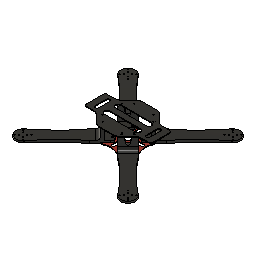
drone-model (Autodesk Fusion 360 design; units mm, degrees)
part number: 2026-04-12-16-53-26-750
Autodesk Fusion 360 part; units mm, degrees
sketch "Sketch1" plane through (0, 0, 0) normal (0, 0, 1) x (1, 0, 0)
  line L0 (-24, 54) -> (24, 54)
  line L1 (54, 24) -> (54, -24)
  line L2 (24, -54) -> (-24, -54)
  line L3 (-54, -24) -> (-54, 24)
  line L4 (-54, 54) -> (54, -54) construction
  line L5 (54, 54) -> (-54, -54) construction
  line L6 (-54, 24) -> (-24, 54)
  line L7 (24, 54) -> (54, 24)
  line L8 (54, -24) -> (24, -54)
  line L9 (-54, -24) -> (-24, -54)
  spline S0 degree 5 poles (-24, 54) (-23.04, 53.5449) (-21.12, 52.6745) (-18.24, 51.4881) (-14.4, 50.1486) (-9.6, 48.9056) (-4.8, 48.1327) (0, 47.868) (4.8, 48.1327) (9.6, 48.9056) (14.4, 50.1486) (18.24, 51.4881) (21.12, 52.6745) (23.04, 53.5449) (24, 54) knots 0 0 0 0 0 0 0.1 0.2 0.3 0.4 0.5 0.6 0.7 0.8 0.9 1 1 1 1 1 1
  spline S1 degree 5 poles (54, 24) (53.5449, 23.04) (52.6745, 21.12) (51.4881, 18.24) (50.1486, 14.4) (48.9056, 9.6) (48.1327, 4.8) (47.868, 0) (48.1327, -4.8) (48.9056, -9.6) (50.1486, -14.4) (51.4881, -18.24) (52.6745, -21.12) (53.5449, -23.04) (54, -24) knots 0 0 0 0 0 0 0.1 0.2 0.3 0.4 0.5 0.6 0.7 0.8 0.9 1 1 1 1 1 1
  spline S2 degree 5 poles (24, -54) (23.04, -53.5449) (21.12, -52.6745) (18.24, -51.4881) (14.4, -50.1486) (9.6, -48.9056) (4.8, -48.1327) (0, -47.868) (-4.8, -48.1327) (-9.6, -48.9056) (-14.4, -50.1486) (-18.24, -51.4881) (-21.12, -52.6745) (-23.04, -53.5449) (-24, -54) knots 0 0 0 0 0 0 0.1 0.2 0.3 0.4 0.5 0.6 0.7 0.8 0.9 1 1 1 1 1 1
  spline S3 degree 5 poles (-54, -24) (-53.5449, -23.04) (-52.6745, -21.12) (-51.4881, -18.24) (-50.1486, -14.4) (-48.9056, -9.6) (-48.1327, -4.8) (-47.868, 0) (-48.1327, 4.8) (-48.9056, 9.6) (-50.1486, 14.4) (-51.4881, 18.24) (-52.6745, 21.12) (-53.5449, 23.04) (-54, 24) knots 0 0 0 0 0 0 0.1 0.2 0.3 0.4 0.5 0.6 0.7 0.8 0.9 1 1 1 1 1 1
  circle A0 centre (-43.2426, 26.2721) radius 1.6
  circle A1 centre (-26.2721, 43.2426) radius 1.6
  circle A2 centre (-26.5578, 15.2441) radius 1.6
  circle A3 centre (-15.2441, 26.5578) radius 1.6
  circle A4 centre (26.2721, -43.2426) radius 1.6
  circle A5 centre (43.2426, -26.2721) radius 1.6
  circle A6 centre (26.5578, -15.2441) radius 1.6
  circle A7 centre (15.2441, -26.5578) radius 1.6
  circle A8 centre (-43.2426, 26.2721) radius 1.6
  circle A9 centre (-26.5578, 15.2441) radius 1.6
  circle A10 centre (-15.2441, 26.5578) radius 1.6
  circle A11 centre (-26.2721, 43.2426) radius 1.6
  line L10 (0, 0) -> (0, 54)
  circle A12 centre (15.2441, 26.5578) radius 1.6
  circle A13 centre (26.2721, 43.2426) radius 1.6
  circle A14 centre (43.2426, 26.2721) radius 1.6
  circle A15 centre (26.5578, 15.2441) radius 1.6
  line L11 (0, 0) -> (0, -54)
  circle A16 centre (-26.5578, -15.2441) radius 1.6
  circle A17 centre (-15.2441, -26.5578) radius 1.6
  circle A18 centre (-26.2721, -43.2426) radius 1.6
  circle A19 centre (-43.2426, -26.2721) radius 1.6
  point P0 (0, 48)
  point P1 (48, 0)
  point P2 (0, -48)
  point P3 (-48, 0)
  dimension "d1" = 108
  dimension "d2" = 108
  dimension "d3" = 30
  dimension "d4" = 30
  dimension "d5" = 30
  dimension "d6" = 30
  dimension "d7" = 30
  dimension "d8" = 30
  dimension "d9" = 30
  dimension "d10" = 30
  dimension "d11" = 6
  dimension "d12" = 6
  dimension "d13" = 6
  dimension "d14" = 6
  dimension "d15" = 3.2
  dimension "d16" = 12
  dimension "d17" = 6
  dimension "d18" = 3.2
  dimension "d19" = 20
  dimension "d20" = 8
  constraint horizontal L0
  constraint perpendicular L0 L1
  constraint parallel L0 L2
  constraint parallel L1 L3
  constraint coincident L4 L10.start
  constraint coincident L5 L10.start
  constraint coincident L10.start L11.start
  constraint coincident L4.start L3
  constraint coincident L4.start L0
  constraint coincident L5.start L0
  constraint coincident L5.start L1
  constraint coincident L4.end L1
  constraint coincident L4.end L2
  constraint coincident L5.end L3
  constraint coincident L5.end L2
  constraint symmetric L4 A0 A1
  constraint symmetric L4 A2 A3
  constraint symmetric L5 A0 A4
  constraint symmetric L5 A1 A5
  constraint symmetric L5 A2 A7
  constraint symmetric L5 A3 A6
  constraint symmetric L4 A0 A11
  constraint symmetric L4 A1 A8
  constraint symmetric L4 A2 A10
  constraint symmetric L4 A3 A9
  constraint midpoint L0 L10.end
  constraint symmetric A8 L10 A14
  constraint symmetric A9 L10 A15
  constraint symmetric A10 L10 A12
  constraint symmetric A11 L10 A13
  constraint midpoint L2 L11.end
  constraint symmetric A4 L11 A18
  constraint symmetric A5 L11 A19
  constraint symmetric A6 L11 A16
  constraint symmetric A7 L11 A17
  measures "d1" distance of L4.end L5.end
  measures "d2" distance of L5.start L4.end
  measures "d3" distance of L4.start L3.end
  measures "d4" distance of L4.start L0.start
  measures "d5" distance of L5.start L0.end
  measures "d6" distance of L5.start L1.start
  measures "d7" distance of L4.end L1.end
  measures "d8" distance of L4.end L2.start
  measures "d9" distance of L5.end L3.start
  measures "d10" distance of L5.end L2.end
  measures "d11" distance of L3 P3
  measures "d12" distance of L0 P0
  measures "d13" distance of L1 P1
  measures "d14" distance of L2 P2
  measures "d15" diameter of A0
  measures "d16" distance of L4 A0.centre
  measures "d17" distance of L6 A0.centre
  measures "d18" diameter of A2
  measures "d19" distance of A0.centre A2.centre
  measures "d20" distance of L4 A2.centre
extrude "Extrude1" add sketch "Sketch1" along normal blind 2 contours L6 L9 S0 S2 S3 L10 L11 | L7 L8 S0 S1 S2 L10 L11 makes body 1
sketch "Sketch2" plane through (0, 0, 2) normal (0, 0, 1) x (-1, 0, 0)
  circle A0 centre (26.2721, 43.2426) radius 1.6
  circle A1 centre (-26.2721, -43.2426) radius 1.6
  circle A2 centre (43.2426, 26.2721) radius 1.6
  circle A3 centre (26.5578, 15.2441) radius 1.6
  circle A4 centre (15.2441, 26.5578) radius 1.6
  circle A5 centre (-15.2441, 26.5578) radius 1.6
  circle A6 centre (-15.2441, -26.5578) radius 1.6
  circle A7 centre (-43.2426, -26.2721) radius 1.6
  circle A8 centre (26.2721, -43.2426) radius 1.6
  circle A9 centre (-43.2426, 26.2721) radius 1.6
  circle A10 centre (15.2441, -26.5578) radius 1.6
  circle A11 centre (43.2426, -26.2721) radius 1.6
  circle A12 centre (-26.5578, 15.2441) radius 1.6
  circle A13 centre (26.5578, -15.2441) radius 1.6
  circle A14 centre (-26.5578, -15.2441) radius 1.6
  circle A15 centre (-26.2721, 43.2426) radius 1.6
  line L0 (54, 24) -> (24, 54)
  spline S0 degree 5 poles (24, 54) (23.04, 53.5449) (21.12, 52.6745) (18.24, 51.4881) (14.4, 50.1486) (9.6, 48.9056) (4.8, 48.1327) (0, 47.868) (-4.8, 48.1327) (-9.6, 48.9056) (-14.4, 50.1486) (-18.24, 51.4881) (-21.12, 52.6745) (-23.04, 53.5449) (-24, 54) knots -1 -1 -1 -1 -1 -1 -0.9 -0.8 -0.7 -0.6 -0.5 -0.4 -0.3 -0.2 -0.1 0 0 0 0 0 0
  line L1 (-24, 54) -> (-54, 24)
  spline S1 degree 5 poles (-54, 24) (-53.5449, 23.04) (-52.6745, 21.12) (-51.4881, 18.24) (-50.1486, 14.4) (-48.9056, 9.6) (-48.1327, 4.8) (-47.868, 0) (-48.1327, -4.8) (-48.9056, -9.6) (-50.1486, -14.4) (-51.4881, -18.24) (-52.6745, -21.12) (-53.5449, -23.04) (-54, -24) knots -1 -1 -1 -1 -1 -1 -0.9 -0.8 -0.7 -0.6 -0.5 -0.4 -0.3 -0.2 -0.1 0 0 0 0 0 0
  line L2 (-54, -24) -> (-24, -54)
  spline S2 degree 5 poles (-24, -54) (-23.04, -53.5449) (-21.12, -52.6745) (-18.24, -51.4881) (-14.4, -50.1486) (-9.6, -48.9056) (-4.8, -48.1327) (0, -47.868) (4.8, -48.1327) (9.6, -48.9056) (14.4, -50.1486) (18.24, -51.4881) (21.12, -52.6745) (23.04, -53.5449) (24, -54) knots -1 -1 -1 -1 -1 -1 -0.9 -0.8 -0.7 -0.6 -0.5 -0.4 -0.3 -0.2 -0.1 0 0 0 0 0 0
  line L3 (24, -54) -> (54, -24)
  spline S3 degree 5 poles (54, -24) (53.5449, -23.04) (52.6745, -21.12) (51.4881, -18.24) (50.1486, -14.4) (48.9056, -9.6) (48.1327, -4.8) (47.868, 0) (48.1327, 4.8) (48.9056, 9.6) (50.1486, 14.4) (51.4881, 18.24) (52.6745, 21.12) (53.5449, 23.04) (54, 24) knots -1 -1 -1 -1 -1 -1 -0.9 -0.8 -0.7 -0.6 -0.5 -0.4 -0.3 -0.2 -0.1 0 0 0 0 0 0
  circle A16 centre (0, 0) radius 12.5
  line L4 (40, 4) -> (20, 4)
  arc A17 (20, 4) -> (20, -4) centre (20, 0) ccw
  line L5 (20, -4) -> (40, -4)
  arc A18 (40, -4) -> (40, 4) centre (40, 0) ccw
  line L6 (40, 0) -> (20, 0) construction
  line L7 (0, -60) -> (0, 60) construction
  line L8 (-20, -4) -> (-40, -4)
  arc A19 (-20, -4) -> (-20, 4) centre (-20, 0) ccw
  line L9 (-40, 4) -> (-20, 4)
  arc A20 (-40, 4) -> (-40, -4) centre (-40, 0) ccw
  line L10 (50, -50) -> (-50, 50) construction
  line L11 (-4, -40) -> (-4, -20)
  arc A21 (4, -20) -> (-4, -20) centre (0, -20) ccw
  line L12 (4, -20) -> (4, -40)
  arc A22 (-4, -40) -> (4, -40) centre (0, -40) ccw
  line L13 (-50, -50) -> (50, 50) construction
  line L14 (4, 40) -> (4, 20)
  arc A23 (4, 40) -> (-4, 40) centre (0, 40) ccw
  line L15 (-4, 20) -> (-4, 40)
  arc A24 (-4, 20) -> (4, 20) centre (0, 20) ccw
  dimension "d23" = 25
  dimension "d24" = 8
  constraint coincident A16.centre origin
  constraint tangent L4 A17
  constraint tangent A17 L5
  constraint parallel L4 L5
  constraint tangent L5 A18
  constraint tangent L4 A18
  constraint horizontal L6
  constraint vertical L7
  constraint symmetric L4.start L7 L9.start
  constraint symmetric L4.end L7 A19.end
  constraint symmetric A17.end L7 L8.start
  constraint symmetric L5.end L7 L8.end
  constraint symmetric A17 L7 A19
  constraint symmetric A18 L7 A20
  constraint symmetric L4.start L10 L11.start
  constraint symmetric L4.end L10 L11.end
  constraint symmetric A17.end L10 A21.start
  constraint symmetric L5.end L10 L12.end
  constraint symmetric A17 L10 A21
  constraint symmetric A18 L10 A22
  constraint perpendicular L0 L13
  constraint symmetric L4.start L13 L14.start
  constraint symmetric L4.end L13 L14.end
  constraint symmetric A17.end L13 L15.start
  constraint symmetric L5.end L13 A23.end
  constraint symmetric A17 L13 A24
  constraint symmetric A18 L13 A23
  measures "d23" diameter of A16
  measures "d24" diameter of A17
extrude "Extrude2" cut sketch "Sketch2" against normal up to surface (2 mm away) contours A16 | L4 A17 L5 A18 | L8 A19 L9 A20 | L11 A21 L12 A22 | L14 A23 L15 A24 bodies 1
fillet "Fillet1" radius 10 8 edges at (-24, 54, 1) (24, 54, 1) (-54, 24, 1) (-54, -24, 1) (-24, -54, 1) (24, -54, 1) (54, -24, 1) (54, 24, 1) on bodies 1
sketch "Sketch3" plane through (0, 0, 2) normal (0, 0, 1) x (-1, 0, 0)
  spline S0 degree 3 poles (-49.2413, -28.7587) (-50.1621, -27.8379) (-50.8942, -26.7461) (-51.8987, -24.3434) (-52.1615, -23.0554) (-52.178, -20.5388) (-51.9647, -19.3329) (-51.5405, -18.1949) knots 0 0 0 0 0.390644 0.390644 0.781289 0.781289 1.145638 1.145638 1.145638 1.145638
  line L0 (-49.2413, -28.7587) -> (-28.7587, -49.2413)
  spline S1 degree 3 poles (-18.1949, -51.5405) (-19.4151, -51.9953) (-20.7124, -52.2074) (-23.3153, -52.1224) (-24.596, -51.8262) (-26.8918, -50.7953) (-27.8999, -50.1001) (-28.7587, -49.2413) knots 0 0 0 0 0.390644 0.390644 0.781289 0.781289 1.145638 1.145638 1.145638 1.145638
  spline S2 degree 5 poles (-18.1949, -51.5405) (-17.4359, -51.2576) (-15.717, -50.6459) (-13.038, -49.7969) (-9.399, -48.8733) (-4.8, -48.1327) (0, -47.868) (4.8, -48.1327) (9.399, -48.8733) (13.038, -49.7969) (15.717, -50.6459) (17.4359, -51.2576) (18.1949, -51.5405) knots -0.879061 -0.879061 -0.879061 -0.879061 -0.879061 -0.879061 -0.8 -0.7 -0.6 -0.5 -0.4 -0.3 -0.2 -0.120939 -0.120939 -0.120939 -0.120939 -0.120939 -0.120939
  spline S3 degree 3 poles (28.7587, -49.2413) (27.8379, -50.1621) (26.7461, -50.8942) (24.3434, -51.8987) (23.0554, -52.1615) (20.5388, -52.178) (19.3329, -51.9647) (18.1949, -51.5405) knots 0 0 0 0 0.390644 0.390644 0.781289 0.781289 1.145638 1.145638 1.145638 1.145638
  line L1 (28.7587, -49.2413) -> (49.2413, -28.7587)
  spline S4 degree 3 poles (51.5405, -18.1949) (51.9953, -19.4151) (52.2074, -20.7124) (52.1224, -23.3153) (51.8262, -24.596) (50.7953, -26.8918) (50.1001, -27.8999) (49.2413, -28.7587) knots 0 0 0 0 0.390644 0.390644 0.781289 0.781289 1.145638 1.145638 1.145638 1.145638
  spline S5 degree 5 poles (51.5405, -18.1949) (51.2576, -17.4359) (50.6459, -15.717) (49.7969, -13.038) (48.8733, -9.399) (48.1327, -4.8) (47.868, 0) (48.1327, 4.8) (48.8733, 9.399) (49.7969, 13.038) (50.6459, 15.717) (51.2576, 17.4359) (51.5405, 18.1949) knots -0.879061 -0.879061 -0.879061 -0.879061 -0.879061 -0.879061 -0.8 -0.7 -0.6 -0.5 -0.4 -0.3 -0.2 -0.120939 -0.120939 -0.120939 -0.120939 -0.120939 -0.120939
  spline S6 degree 3 poles (49.2413, 28.7587) (50.1621, 27.8379) (50.8942, 26.7461) (51.8987, 24.3434) (52.1615, 23.0554) (52.178, 20.5388) (51.9647, 19.3329) (51.5405, 18.1949) knots 0 0 0 0 0.390644 0.390644 0.781289 0.781289 1.145638 1.145638 1.145638 1.145638
  line L2 (49.2413, 28.7587) -> (28.7587, 49.2413)
  spline S7 degree 3 poles (18.1949, 51.5405) (19.4151, 51.9953) (20.7124, 52.2074) (23.3153, 52.1224) (24.596, 51.8262) (26.8918, 50.7953) (27.8999, 50.1001) (28.7587, 49.2413) knots 0 0 0 0 0.390644 0.390644 0.781289 0.781289 1.145638 1.145638 1.145638 1.145638
  spline S8 degree 5 poles (18.1949, 51.5405) (17.4359, 51.2576) (15.717, 50.6459) (13.038, 49.7969) (9.399, 48.8733) (4.8, 48.1327) (0, 47.868) (-4.8, 48.1327) (-9.399, 48.8733) (-13.038, 49.7969) (-15.717, 50.6459) (-17.4359, 51.2576) (-18.1949, 51.5405) knots -0.879061 -0.879061 -0.879061 -0.879061 -0.879061 -0.879061 -0.8 -0.7 -0.6 -0.5 -0.4 -0.3 -0.2 -0.120939 -0.120939 -0.120939 -0.120939 -0.120939 -0.120939
  spline S9 degree 3 poles (-28.7587, 49.2413) (-27.8379, 50.1621) (-26.7461, 50.8942) (-24.3434, 51.8987) (-23.0554, 52.1615) (-20.5388, 52.178) (-19.3329, 51.9647) (-18.1949, 51.5405) knots 0 0 0 0 0.390644 0.390644 0.781289 0.781289 1.145638 1.145638 1.145638 1.145638
  line L3 (-28.7587, 49.2413) -> (-49.2413, 28.7587)
  spline S10 degree 3 poles (-51.5405, 18.1949) (-51.9953, 19.4151) (-52.2074, 20.7124) (-52.1224, 23.3153) (-51.8262, 24.596) (-50.7953, 26.8918) (-50.1001, 27.8999) (-49.2413, 28.7587) knots 0 0 0 0 0.390644 0.390644 0.781289 0.781289 1.145638 1.145638 1.145638 1.145638
  spline S11 degree 5 poles (-51.5405, 18.1949) (-51.2576, 17.4359) (-50.6459, 15.717) (-49.7969, 13.038) (-48.8733, 9.399) (-48.1327, 4.8) (-47.868, 0) (-48.1327, -4.8) (-48.8733, -9.399) (-49.7969, -13.038) (-50.6459, -15.717) (-51.2576, -17.4359) (-51.5405, -18.1949) knots -0.879061 -0.879061 -0.879061 -0.879061 -0.879061 -0.879061 -0.8 -0.7 -0.6 -0.5 -0.4 -0.3 -0.2 -0.120939 -0.120939 -0.120939 -0.120939 -0.120939 -0.120939
  line L4 (40, -4) -> (20, -4)
  arc A0 (20, 4) -> (20, -4) centre (20, 0) ccw
  line L5 (20, 4) -> (40, 4)
  arc A1 (40, -4) -> (40, 4) centre (40, 0) ccw
  circle A2 centre (0, 0) radius 12.5
  line L6 (4, -20) -> (4, -40)
  arc A3 (-4, -40) -> (4, -40) centre (0, -40) ccw
  line L7 (-4, -40) -> (-4, -20)
  arc A4 (4, -20) -> (-4, -20) centre (0, -20) ccw
  line L8 (-20, -4) -> (-40, -4)
  arc A5 (-40, 4) -> (-40, -4) centre (-40, 0) ccw
  line L9 (-40, 4) -> (-20, 4)
  arc A6 (-20, -4) -> (-20, 4) centre (-20, 0) ccw
  line L10 (4, 40) -> (4, 20)
  arc A7 (-4, 20) -> (4, 20) centre (0, 20) ccw
  line L11 (-4, 20) -> (-4, 40)
  arc A8 (4, 40) -> (-4, 40) centre (0, 40) ccw
  circle A9 centre (26.2721, 43.2426) radius 1.6
  circle A10 centre (-26.2721, -43.2426) radius 1.6
  circle A11 centre (43.2426, 26.2721) radius 1.6
  circle A12 centre (26.5578, 15.2441) radius 1.6
  circle A13 centre (15.2441, 26.5578) radius 1.6
  circle A14 centre (-15.2441, 26.5578) radius 1.6
  circle A15 centre (-15.2441, -26.5578) radius 1.6
  circle A16 centre (-43.2426, -26.2721) radius 1.6
  circle A17 centre (26.2721, -43.2426) radius 1.6
  circle A18 centre (-43.2426, 26.2721) radius 1.6
  circle A19 centre (15.2441, -26.5578) radius 1.6
  circle A20 centre (43.2426, -26.2721) radius 1.6
  circle A21 centre (-26.5578, 15.2441) radius 1.6
  circle A22 centre (26.5578, -15.2441) radius 1.6
  circle A23 centre (-26.5578, -15.2441) radius 1.6
  circle A24 centre (-26.2721, 43.2426) radius 1.6
  circle A25 centre (43.2426, -26.2721) radius 2.5
  circle A26 centre (26.5578, -15.2441) radius 2.5
  circle A27 centre (26.2721, -43.2426) radius 2.5
  circle A28 centre (15.2441, -26.5578) radius 2.5
  line L12 (0, 0) -> (176.7767, -176.7767) construction
  line L13 (0, 0) -> (250, 0) construction
  line L14 (53.1421, -24.8579) -> (24.8579, -53.1421)
  line L15 (24.8579, -53.1421) -> (9.3015, -37.5858)
  line L16 (9.3015, -26.2721) -> (26.2721, -9.3015)
  line L17 (37.5858, -9.3015) -> (53.1421, -24.8579)
  arc A29 (37.5858, -9.3015) -> (26.2721, -9.3015) centre (31.9289, -14.9584) ccw
  arc A30 (9.3015, -26.2721) -> (9.3015, -37.5858) centre (14.9584, -31.9289) ccw
  line L18 (53.1421, -24.8579) -> (221.1421, -24.8579) construction
  spline S12 degree 5 poles (157.3028, -129.0185) (154.9274, -127.1077) (150.2243, -123.2951) (143.3125, -117.6026) (134.3873, -110.0668) (123.7498, -100.7436) (113.6845, -91.5269) (104.2498, -82.4275) (95.4955, -73.4547) (87.427, -64.6096) (80.0061, -55.885) (74.5517, -48.995) (70.7161, -43.8751) (68.2706, -40.4825) (67.0757, -38.7914) knots 0 0 0 0 0 0 0.1 0.2 0.3 0.4 0.5 0.6 0.7 0.8 0.9 1 1 1 1 1 1
  line L19 (53.1421, -24.8579) -> (67.0757, -38.7914)
  line L20 (157.3028, -129.0185) -> (157.7598, -129.4756)
  arc A31 (127.2471, -155.1069) -> (155.1069, -127.2471) centre (143.6177, -143.6177) ccw
  spline S13 degree 5 poles (129.0185, -157.3028) (127.1077, -154.9274) (123.2951, -150.2243) (117.6026, -143.3125) (110.0668, -134.3873) (100.7436, -123.7498) (91.5269, -113.6845) (82.4275, -104.2498) (73.4547, -95.4955) (64.6096, -87.427) (55.885, -80.0061) (48.995, -74.5517) (43.8751, -70.7161) (40.4825, -68.2706) (38.7914, -67.0757) knots 0 0 0 0 0 0 0.1 0.2 0.3 0.4 0.5 0.6 0.7 0.8 0.9 1 1 1 1 1 1
  line L21 (168.7702, -138.2431) -> (145.8353, -119.794)
  line L22 (74.1541, -48.8094) -> (59.9973, -28.7735)
  line L23 (138.2431, -168.7702) -> (119.794, -145.8353)
  line L24 (48.8094, -74.1541) -> (28.7735, -59.9973)
  line L25 (38.7914, -67.0757) -> (24.8579, -53.1421)
  line L26 (143.6177, -143.6177) -> (151, -151) construction
  line L27 (143.6177, -143.6177) -> (155.1789, -155.1789) construction
  circle A32 centre (155.1789, -155.1789) radius 1.6
  circle A33 centre (149.1685, -149.1685) radius 1.6
  line L28 (143.6177, -143.6177) -> (161, -143.6177) construction
  line L29 (143.6177, -143.6177) -> (143.6177, -158) construction
  line L30 (143.6177, -143.6177) -> (143.6177, -130) construction
  line L31 (143.6177, -143.6177) -> (130, -143.6177) construction
  circle A34 centre (132.0565, -155.1789) radius 1.6
  circle A35 centre (138.0669, -149.1685) radius 1.6
  circle A36 centre (138.0669, -138.0669) radius 1.6
  circle A37 centre (132.0565, -132.0565) radius 1.6
  circle A38 centre (149.1685, -138.0669) radius 1.6
  circle A39 centre (155.1789, -132.0565) radius 1.6
  point P0 (31.9289, -3.6447)
  point P1 (100, -78)
  point P2 (78, -100)
  dimension "d29" = 5
  dimension "d30" = 5
  dimension "d31" = 5
  dimension "d32" = 5
  dimension "d33" = 45
  dimension "d34" = 250
  dimension "d35" = 40
  dimension "d36" = 20
  dimension "d37" = 30
  dimension "d38" = 8
  dimension "d39" = 45
  dimension "d42" = 40
  dimension "d43" = 16.35
  dimension "d44" = 3.2
  dimension "d45" = 3.2
  dimension "d46" = 7.85
  constraint concentric A20 A25
  constraint concentric A22 A26
  constraint concentric A17 A27
  constraint concentric A19 A28
  constraint horizontal L13
  constraint coincident A2.centre L12.start
  constraint perpendicular L14 L15
  constraint perpendicular L12 L16
  constraint parallel L1 L14
  constraint parallel L15 L17
  constraint coincident L1 L14.start
  constraint coincident P0 L17
  constraint coincident P0 L16
  constraint tangent L17 A29
  constraint tangent L16 A29
  constraint tangent L16 A30
  constraint tangent L15 A30
  constraint equal A29 A30
  constraint horizontal L18
  constraint coincident L12 A31.centre
  constraint collinear L19 L20
  constraint coincident L20.end A31
  constraint coincident S12 A31.end
  constraint midpoint S12.start L21
  constraint midpoint S12.end L22
  constraint symmetric L12 S12.start S13.start
  constraint symmetric L12 P1 P2
  constraint symmetric L12 S12.end S13.end
  constraint symmetric L12 L21.start L23.start
  constraint symmetric L12 L21.end L23.end
  constraint symmetric L12 L22.start L24.start
  constraint symmetric L12 L22.end L24.end
  constraint coincident S13 A31.start
  constraint coincident A31.centre L26.start
  constraint coincident L12 L26.end
  constraint parallel L26 L27
  constraint coincident L27.end A32.centre
  constraint coincident L27 A33.centre
  constraint horizontal L28
  constraint perpendicular L28 L29
  constraint parallel L29 L30
  constraint perpendicular L30 L31
  constraint symmetric A32 L29 A34
  constraint symmetric A33 L29 A35
  constraint symmetric A32 L31 A39
  constraint symmetric A33 L31 A38
  constraint symmetric L31 A34 A37
  constraint symmetric L31 A35 A36
  measures "d29" diameter of A25
  measures "d30" diameter of A26
  measures "d31" diameter of A27
  measures "d32" diameter of A28
  measures "d33" angle of L12 L13
  measures "d34" distance of A2.centre L12.end
  measures "d35" distance of L14.start L14.end
  measures "d36" distance of L12 L17
  measures "d37" distance of L14.start P0
  measures "d38" radius of A29
  measures "d39" angle of L18 L19
  measures "d42" diameter of A31
  measures "d43" distance of A31.centre L27.end
  measures "d44" diameter of A32
  measures "d45" diameter of A33
  measures "d46" distance of A31.centre A33.centre
extrude "Extrude3" add sketch "Sketch3" along normal blind 5 separate body contours S3 L1 S4 L14 L15 L16 L17 A29 A30 | S3 L14 L15 | L1 L14 S12 L19 A31 S13 L25 | S4 L14 L17 makes body 2
sketch "Sketch4" plane through (0, 0, 7) normal (0, 0, 1) x (-1, 0, 0)
  circle A0 centre (132.0565, -155.1789) radius 1.6
  circle A1 centre (26.2721, -43.2426) radius 2.5
  circle A2 centre (43.2426, -26.2721) radius 2.5
  circle A3 centre (138.0669, -149.1685) radius 1.6
  circle A4 centre (149.1685, -149.1685) radius 1.6
  circle A5 centre (149.1685, -138.0669) radius 1.6
  circle A6 centre (155.1789, -132.0565) radius 1.6
  circle A7 centre (26.5578, -15.2441) radius 2.5
  circle A8 centre (155.1789, -155.1789) radius 1.6
  circle A9 centre (132.0565, -132.0565) radius 1.6
  circle A10 centre (138.0669, -138.0669) radius 1.6
  circle A11 centre (15.2441, -26.5578) radius 2.5
  arc A12 (128.9275, -157.1896) -> (157.1896, -128.9275) centre (143.6177, -143.6177) ccw
  spline S0 degree 5 poles (157.1896, -128.9275) (156.7716, -128.5911) (156.3543, -128.2549) (155.9378, -127.9188) (155.522, -127.5829) (155.1069, -127.2471) knots 0.000953 0.000953 0.000953 0.000953 0.000953 0.000953 0.018558 0.018558 0.018558 0.018558 0.018558 0.018558
  spline S1 degree 5 poles (155.1069, -127.2471) (153.1868, -125.6936) (148.9441, -122.2392) (142.4853, -116.9036) (133.9925, -109.7208) (123.7498, -100.7436) (113.6845, -91.5269) (104.2498, -82.4275) (95.4955, -73.4547) (87.427, -64.6096) (80.0061, -55.885) (74.5517, -48.995) (70.7161, -43.8751) (68.2706, -40.4825) (67.0757, -38.7914) knots 0.018558 0.018558 0.018558 0.018558 0.018558 0.018558 0.1 0.2 0.3 0.4 0.5 0.6 0.7 0.8 0.9 1 1 1 1 1 1
  line L0 (67.0757, -38.7914) -> (37.5858, -9.3015)
  arc A13 (37.5858, -9.3015) -> (26.2721, -9.3015) centre (31.9289, -14.9584) ccw
  line L1 (26.2721, -9.3015) -> (9.3015, -26.2721)
  arc A14 (9.3015, -26.2721) -> (9.3015, -37.5858) centre (14.9584, -31.9289) ccw
  line L2 (9.3015, -37.5858) -> (38.7914, -67.0757)
  spline S2 degree 5 poles (38.7914, -67.0757) (40.4825, -68.2706) (43.8751, -70.7161) (48.995, -74.5517) (55.885, -80.0061) (64.6096, -87.427) (73.4547, -95.4955) (82.4275, -104.2498) (91.5269, -113.6845) (100.7436, -123.7498) (109.7208, -133.9925) (116.9036, -142.4853) (122.2392, -148.9441) (125.6936, -153.1868) (127.2471, -155.1069) knots -1 -1 -1 -1 -1 -1 -0.9 -0.8 -0.7 -0.6 -0.5 -0.4 -0.3 -0.2 -0.1 -0.018558 -0.018558 -0.018558 -0.018558 -0.018558 -0.018558
  spline S3 degree 5 poles (127.2471, -155.1069) (127.5829, -155.522) (127.9188, -155.9378) (128.2549, -156.3543) (128.5911, -156.7716) (128.9275, -157.1896) knots -0.018558 -0.018558 -0.018558 -0.018558 -0.018558 -0.018558 -0.000953 -0.000953 -0.000953 -0.000953 -0.000953 -0.000953
  circle A15 centre (26.2721, -43.2426) radius 2.5
  circle A16 centre (43.2426, -26.2721) radius 2.5
  line L3 (45.88, -17.5957) -> (85.88, -17.5957) construction
  circle A17 centre (43.2426, -26.2721) radius 2.5
  line L4 (51.7279, -23.4437) -> (23.4437, -51.7279)
  line L5 (17.7868, -46.0711) -> (46.0711, -17.7868)
  dimension "d49" = 5
  dimension "d51" = 5
  dimension "d52" = 8
  dimension "d53" = 4
  constraint concentric A1 A15
  constraint concentric A2 A16
  constraint horizontal L3
  constraint coincident L0 L3.start
  constraint concentric A16 A17
  constraint coincident L0 L4.start
  constraint coincident L2 L4.end
  constraint perpendicular L2 L4
  constraint coincident L2 L5.start
  constraint coincident L0 L5.end
  constraint perpendicular L0 L5
  measures "d49" diameter of A15
  measures "d51" diameter of A17
  measures "d52" distance of L4 L5
  measures "d53" distance of A2.centre L4
extrude "Extrude4" add sketch "Sketch4" along normal blind 37 contours L0 L2 L4 L5 bodies 2
fillet "Fillet2" radius 5 2 edges at (-48.8995, 20.6152, 44) (-20.6152, 48.8995, 44) on bodies 2
sketch "Sketch5" plane through (-31.9289, 31.9289, 0) normal (0.707107, -0.707107, 0) x (0.707107, 0.707107, 0)
  arc A0 (20, 39) -> (15, 44) centre (15, 39) ccw
  line L0 (15, 44) -> (-15, 44)
  arc A1 (-15, 44) -> (-20, 39) centre (-15, 39) ccw
  line L1 (-20, 39) -> (-20, 7)
  line L2 (-20, 7) -> (20, 7)
  line L3 (20, 7) -> (20, 39)
  line L4 (0, 44) -> (0, 7) construction
  line L5 (-8, 44) -> (-4, 18.0376)
  line L6 (-4, 18.0376) -> (0, 18.0376)
  line L7 (8, 44) -> (4, 18.0376)
  line L8 (4, 18.0376) -> (0, 18.0376)
  line L9 (-8, 44) -> (8, 44)
  dimension "d58" = 8
  dimension "d59" = 4
  constraint midpoint L0 L4.start
  constraint midpoint L2 L4.end
  constraint coincident L0 L5.start
  constraint coincident L4 L6.end
  constraint perpendicular L4 L6
  constraint symmetric L4 L5.start L7.start
  constraint symmetric L4 L5.end L7.end
  constraint symmetric L4 L6.end L8.end
  measures "d58" distance of L4.start L5.start
  measures "d59" distance of L5.end L6.end
extrude "Extrude5" cut sketch "Sketch5" against normal blind 10 contours L0 L5 L6 L7 L8 L9 bodies 2
fillet "Fillet3" radius 2 2 edges at (-40.4142, 29.1005, 44) (-29.1005, 40.4142, 44) on bodies 2
fillet "Fillet4" radius 5 2 edges at (-31.9289, 37.5858, 18.0376) (-37.5858, 31.9289, 18.0376) on bodies 2
sketch "Sketch6" plane through (0, 0, 2) normal (0, 0, -1) x (1, 0, 0)
  circle A0 centre (-132.0565, -155.1789) radius 1.6
  circle A1 centre (-26.2721, -43.2426) radius 2.5
  circle A2 centre (-43.2426, -26.2721) radius 2.5
  circle A3 centre (-138.0669, -149.1685) radius 1.6
  circle A4 centre (-149.1685, -149.1685) radius 1.6
  circle A5 centre (-149.1685, -138.0669) radius 1.6
  circle A6 centre (-155.1789, -132.0565) radius 1.6
  circle A7 centre (-26.5578, -15.2441) radius 2.5
  circle A8 centre (-155.1789, -155.1789) radius 1.6
  circle A9 centre (-132.0565, -132.0565) radius 1.6
  circle A10 centre (-138.0669, -138.0669) radius 1.6
  circle A11 centre (-15.2441, -26.5578) radius 2.5
  arc A12 (-157.1896, -128.9275) -> (-128.9275, -157.1896) centre (-143.6177, -143.6177) ccw
  spline S0 degree 5 poles (-128.9275, -157.1896) (-128.5911, -156.7716) (-128.2549, -156.3543) (-127.9188, -155.9378) (-127.5829, -155.522) (-127.2471, -155.1069) knots 0.000953 0.000953 0.000953 0.000953 0.000953 0.000953 0.018558 0.018558 0.018558 0.018558 0.018558 0.018558
  spline S1 degree 5 poles (-127.2471, -155.1069) (-125.6936, -153.1868) (-122.2392, -148.9441) (-116.9036, -142.4853) (-109.7208, -133.9925) (-100.7436, -123.7498) (-91.5269, -113.6845) (-82.4275, -104.2498) (-73.4547, -95.4955) (-64.6096, -87.427) (-55.885, -80.0061) (-48.995, -74.5517) (-43.8751, -70.7161) (-40.4825, -68.2706) (-38.7914, -67.0757) knots 0.018558 0.018558 0.018558 0.018558 0.018558 0.018558 0.1 0.2 0.3 0.4 0.5 0.6 0.7 0.8 0.9 1 1 1 1 1 1
  line L0 (-38.7914, -67.0757) -> (-9.3015, -37.5858)
  arc A13 (-9.3015, -37.5858) -> (-9.3015, -26.2721) centre (-14.9584, -31.9289) ccw
  line L1 (-9.3015, -26.2721) -> (-26.2721, -9.3015)
  arc A14 (-26.2721, -9.3015) -> (-37.5858, -9.3015) centre (-31.9289, -14.9584) ccw
  line L2 (-37.5858, -9.3015) -> (-67.0757, -38.7914)
  spline S2 degree 5 poles (-155.1069, -127.2471) (-153.1868, -125.6936) (-148.9441, -122.2392) (-142.4853, -116.9036) (-133.9925, -109.7208) (-123.7498, -100.7436) (-113.6845, -91.5269) (-104.2498, -82.4275) (-95.4955, -73.4547) (-87.427, -64.6096) (-80.0061, -55.885) (-74.5517, -48.995) (-70.7161, -43.8751) (-68.2706, -40.4825) (-67.0757, -38.7914) knots 0.018558 0.018558 0.018558 0.018558 0.018558 0.018558 0.1 0.2 0.3 0.4 0.5 0.6 0.7 0.8 0.9 1 1 1 1 1 1
  spline S3 degree 5 poles (-157.1896, -128.9275) (-156.7716, -128.5911) (-156.3543, -128.2549) (-155.9378, -127.9188) (-155.522, -127.5829) (-155.1069, -127.2471) knots 0.000953 0.000953 0.000953 0.000953 0.000953 0.000953 0.018558 0.018558 0.018558 0.018558 0.018558 0.018558
  circle A15 centre (-155.1789, -155.1789) radius 1.6
  circle A16 centre (-149.1685, -149.1685) radius 1.6
  circle A17 centre (-149.1685, -138.0669) radius 1.6
  circle A18 centre (-155.1789, -132.0565) radius 1.6
  circle A19 centre (-138.0669, -149.1685) radius 1.6
  circle A20 centre (-132.0565, -155.1789) radius 1.6
  circle A21 centre (-138.0669, -138.0669) radius 1.6
  circle A22 centre (-132.0565, -132.0565) radius 1.6
  arc A23 (-157.1896, -128.9275) -> (-128.9275, -157.1896) centre (-143.6177, -143.6177) ccw
  spline S4 degree 5 poles (-127.2471, -155.1069) (-125.6936, -153.1868) (-122.2392, -148.9441) (-116.9036, -142.4853) (-109.7208, -133.9925) (-100.7436, -123.7498) (-91.5269, -113.6845) (-82.4275, -104.2498) (-73.4547, -95.4955) (-64.6096, -87.427) (-55.885, -80.0061) (-48.995, -74.5517) (-43.8751, -70.7161) (-40.4825, -68.2706) (-38.7914, -67.0757) knots 0.018558 0.018558 0.018558 0.018558 0.018558 0.018558 0.1 0.2 0.3 0.4 0.5 0.6 0.7 0.8 0.9 1 1 1 1 1 1
  spline S5 degree 5 poles (-155.1069, -127.2471) (-153.1868, -125.6936) (-148.9441, -122.2392) (-142.4853, -116.9036) (-133.9925, -109.7208) (-123.7498, -100.7436) (-113.6845, -91.5269) (-104.2498, -82.4275) (-95.4955, -73.4547) (-87.427, -64.6096) (-80.0061, -55.885) (-74.5517, -48.995) (-70.7161, -43.8751) (-68.2706, -40.4825) (-67.0757, -38.7914) knots 0.018558 0.018558 0.018558 0.018558 0.018558 0.018558 0.1 0.2 0.3 0.4 0.5 0.6 0.7 0.8 0.9 1 1 1 1 1 1
  line L3 (-37.5858, -9.3015) -> (-67.0757, -38.7914)
  line L4 (-38.7914, -67.0757) -> (-9.3015, -37.5858)
  line L5 (-155.1069, -127.2471) -> (-153.1868, -125.6936) construction
  line L6 (-153.1868, -125.6936) -> (-148.9441, -122.2392) construction
  line L7 (-148.9441, -122.2392) -> (-142.4853, -116.9036) construction
  line L8 (-142.4853, -116.9036) -> (-133.9925, -109.7208) construction
  line L9 (-133.9925, -109.7208) -> (-123.7498, -100.7436) construction
  line L10 (-123.7498, -100.7436) -> (-113.6845, -91.5269) construction
  line L11 (-113.6845, -91.5269) -> (-104.2498, -82.4275) construction
  line L12 (-104.2498, -82.4275) -> (-95.4955, -73.4547) construction
  line L13 (-95.4955, -73.4547) -> (-87.427, -64.6096) construction
  line L14 (-87.427, -64.6096) -> (-80.0061, -55.885) construction
  line L15 (-80.0061, -55.885) -> (-74.5517, -48.995) construction
  line L16 (-74.5517, -48.995) -> (-70.7161, -43.8751) construction
  line L17 (-70.7161, -43.8751) -> (-68.2706, -40.4825) construction
  line L18 (-68.2706, -40.4825) -> (-67.0757, -38.7914) construction
  line L19 (-127.2471, -155.1069) -> (-125.6936, -153.1868) construction
  line L20 (-125.6936, -153.1868) -> (-122.2392, -148.9441) construction
  line L21 (-122.2392, -148.9441) -> (-116.9036, -142.4853) construction
  line L22 (-116.9036, -142.4853) -> (-109.7208, -133.9925) construction
  line L23 (-109.7208, -133.9925) -> (-100.7436, -123.7498) construction
  line L24 (-100.7436, -123.7498) -> (-91.5269, -113.6845) construction
  line L25 (-91.5269, -113.6845) -> (-82.4275, -104.2498) construction
  line L26 (-82.4275, -104.2498) -> (-73.4547, -95.4955) construction
  line L27 (-73.4547, -95.4955) -> (-64.6096, -87.427) construction
  line L28 (-64.6096, -87.427) -> (-55.885, -80.0061) construction
  line L29 (-55.885, -80.0061) -> (-48.995, -74.5517) construction
  line L30 (-48.995, -74.5517) -> (-43.8751, -70.7161) construction
  line L31 (-43.8751, -70.7161) -> (-40.4825, -68.2706) construction
  line L32 (-40.4825, -68.2706) -> (-38.7914, -67.0757) construction
  line L33 (-49.2413, -28.7587) -> (-28.7587, -49.2413)
  spline S6 degree 3 poles (-23.6846, -51.9688) (-24.4055, -51.8219) (-25.1096, -51.5955) (-26.8918, -50.7953) (-27.8999, -50.1001) (-28.7587, -49.2413) knots 0.559552 0.559552 0.559552 0.559552 0.781289 0.781289 1.145638 1.145638 1.145638 1.145638
  line L34 (-23.6846, -51.9688) -> (-24.4055, -51.8219) construction
  line L35 (-24.4055, -51.8219) -> (-25.1096, -51.5955) construction
  line L36 (-25.1096, -51.5955) -> (-26.8918, -50.7953) construction
  line L37 (-26.8918, -50.7953) -> (-27.8999, -50.1001) construction
  line L38 (-27.8999, -50.1001) -> (-28.7587, -49.2413) construction
  spline S7 degree 3 poles (-49.2413, -28.7587) (-50.1621, -27.8379) (-50.8942, -26.7461) (-51.6479, -24.9434) (-51.8393, -24.3203) (-51.9688, -23.6846) knots 0 0 0 0 0.390644 0.390644 0.586193 0.586193 0.586193 0.586193
  line L39 (-49.2413, -28.7587) -> (-50.1621, -27.8379) construction
  line L40 (-50.1621, -27.8379) -> (-50.8942, -26.7461) construction
  line L41 (-50.8942, -26.7461) -> (-51.6479, -24.9434) construction
  line L42 (-51.6479, -24.9434) -> (-51.8393, -24.3203) construction
  line L43 (-51.8393, -24.3203) -> (-51.9688, -23.6846) construction
  constraint coincident L0 S6.start
  constraint coincident L2 S7.end
extrude "Extrude6" add sketch "Sketch6" along normal blind 2 separate body contours A12 S0 S1 L0 L2 S2 S3 A23 S4 S5 L3 L4 L33 S6 S7 makes body 3
combine "Combine1" operation add target body 3 tool bodies 2
sketch "Sketch7" plane through (0, 0, 0) normal (0, 0, -1) x (1, 0, 0)
  circle A0 centre (-149.1685, -149.1685) radius 1.6
  circle A1 centre (-132.0565, -132.0565) radius 1.6
  circle A2 centre (-138.0669, -149.1685) radius 1.6
  circle A3 centre (-138.0669, -138.0669) radius 1.6
  circle A4 centre (-132.0565, -155.1789) radius 1.6
  circle A5 centre (-155.1789, -155.1789) radius 1.6
  circle A6 centre (-155.1789, -132.0565) radius 1.6
  circle A7 centre (-149.1685, -138.0669) radius 1.6
  arc A8 (-157.1896, -128.9275) -> (-128.9275, -157.1896) centre (-143.6177, -143.6177) ccw
  spline S0 degree 5 poles (-128.9275, -157.1896) (-128.5911, -156.7716) (-128.2549, -156.3543) (-127.9188, -155.9378) (-127.5829, -155.522) (-127.2471, -155.1069) knots 0.000953 0.000953 0.000953 0.000953 0.000953 0.000953 0.018558 0.018558 0.018558 0.018558 0.018558 0.018558
  spline S1 degree 5 poles (-127.2471, -155.1069) (-125.6936, -153.1868) (-122.2392, -148.9441) (-116.9036, -142.4853) (-109.7208, -133.9925) (-100.7436, -123.7498) (-91.5269, -113.6845) (-82.4275, -104.2498) (-73.4547, -95.4955) (-64.6096, -87.427) (-55.885, -80.0061) (-48.995, -74.5517) (-43.8751, -70.7161) (-40.4825, -68.2706) (-38.7914, -67.0757) knots 0.018558 0.018558 0.018558 0.018558 0.018558 0.018558 0.1 0.2 0.3 0.4 0.5 0.6 0.7 0.8 0.9 1 1 1 1 1 1
  line L0 (-38.7914, -67.0757) -> (-23.6846, -51.9688)
  spline S2 degree 3 poles (-23.6846, -51.9688) (-24.4055, -51.8219) (-25.1096, -51.5955) (-26.8918, -50.7953) (-27.8999, -50.1001) (-28.7587, -49.2413) knots 0.559552 0.559552 0.559552 0.559552 0.781289 0.781289 1.145638 1.145638 1.145638 1.145638
  line L1 (-28.7587, -49.2413) -> (-49.2413, -28.7587)
  spline S3 degree 3 poles (-49.2413, -28.7587) (-50.1621, -27.8379) (-50.8942, -26.7461) (-51.6479, -24.9434) (-51.8393, -24.3203) (-51.9688, -23.6846) knots 0 0 0 0 0.390644 0.390644 0.586193 0.586193 0.586193 0.586193
  line L2 (-51.9688, -23.6846) -> (-67.0757, -38.7914)
  spline S4 degree 5 poles (-67.0757, -38.7914) (-68.2706, -40.4825) (-70.7161, -43.8751) (-74.5517, -48.995) (-80.0061, -55.885) (-87.427, -64.6096) (-95.4955, -73.4547) (-104.2498, -82.4275) (-113.6845, -91.5269) (-123.7498, -100.7436) (-133.9925, -109.7208) (-142.4853, -116.9036) (-148.9441, -122.2392) (-153.1868, -125.6936) (-155.1069, -127.2471) knots -1 -1 -1 -1 -1 -1 -0.9 -0.8 -0.7 -0.6 -0.5 -0.4 -0.3 -0.2 -0.1 -0.018558 -0.018558 -0.018558 -0.018558 -0.018558 -0.018558
  spline S5 degree 5 poles (-155.1069, -127.2471) (-155.522, -127.5829) (-155.9378, -127.9188) (-156.3543, -128.2549) (-156.7716, -128.5911) (-157.1896, -128.9275) knots -0.018558 -0.018558 -0.018558 -0.018558 -0.018558 -0.018558 -0.000953 -0.000953 -0.000953 -0.000953 -0.000953 -0.000953
  circle A9 centre (-143.6177, -143.6177) radius 20
  dimension "d68" = 40
  constraint concentric A8 A9
  measures "d68" diameter of A9
extrude "Extrude7" cut sketch "Sketch7" against normal blind 2 contours A8 S0 S5 A9 bodies 3
fillet "Fillet5" radius 50 1 edges at (-129.4756, 129.4756, 0) on bodies 3
mirror "Mirror1" about plane through (0, 0, 0) normal (0, 1, 0) of bodies 3 makes body 4
mirror "Mirror2" about plane through (0, 0, 0) normal (1, 0, 0) of bodies 4 3 makes body 5 at (108.6736, 108.7191, 7) makes body 6 at (108.6736, -108.7191, 7)
sketch "Sketch8" plane through (0, 0, 44) normal (0, 0, 1) x (-1, 0, 0)
  line L0 (-42.3452, 28.6054) -> (-44.4557, 30.7159)
  line L1 (-44.4557, 30.7159) -> (-48.1924, 26.9792)
  line L2 (-48.1924, 26.9792) -> (-42.5355, 21.3223)
  line L3 (-42.5355, 21.3223) -> (-38.7988, 25.0591)
  line L4 (-38.7988, 25.0591) -> (-40.9093, 27.1696)
  arc A0 (-42.3452, 28.6054) -> (-40.9093, 27.1696) centre (-43.2426, 26.2721) ccw
  line L5 (18.7124, 59) -> (-27, 59)
  line L6 (-91, 23.5) -> (-91, -23.5)
  line L7 (-18.7124, -59) -> (18.7124, -59)
  line L8 (91, -23.5) -> (91, 23.5)
  line L9 (91, 59) -> (-91, -59) construction
  line L10 (-91, 59) -> (91, -59) construction
  circle A1 centre (43.2426, -26.2721) radius 1.6
  circle A2 centre (26.2721, -43.2426) radius 1.6
  circle A3 centre (-26.2721, -43.2426) radius 1.6
  circle A4 centre (-43.2426, -26.2721) radius 1.6
  circle A5 centre (-43.2426, 26.2721) radius 1.6
  circle A6 centre (-26.2721, 43.2426) radius 1.6
  circle A7 centre (43.2426, 26.2721) radius 1.6
  circle A8 centre (26.2721, 43.2426) radius 1.6
  line L11 (91, 0) -> (91, -28.5)
  line L12 (86, -28.5) -> (65.7702, -28.5)
  line L13 (51.624, -34.3619) -> (32.8586, -53.1381)
  line L14 (0, -70) -> (0, 80) construction
  line L15 (-51.624, -34.3619) -> (-32.8586, -53.1381)
  line L16 (-86, -28.5) -> (-65.7702, -28.5)
  line L17 (-110, 0) -> (100, 0) construction
  line L18 (51.624, 34.3619) -> (32.8586, 53.1381)
  line L19 (86, 28.5) -> (65.7702, 28.5)
  line L20 (-18.7124, 59) -> (27, 59)
  line L21 (-51.624, 34.3619) -> (-32.8586, 53.1381)
  line L22 (-86, 28.5) -> (-65.7702, 28.5)
  arc A9 (86, -28.5) -> (91, -23.5) centre (86, -23.5) ccw
  arc A10 (91, 23.5) -> (86, 28.5) centre (86, 23.5) ccw
  arc A11 (-91, -23.5) -> (-86, -28.5) centre (-86, -23.5) ccw
  arc A12 (-86, 28.5) -> (-91, 23.5) centre (-86, 23.5) ccw
  arc A13 (-51.624, -34.3619) -> (-65.7702, -28.5) centre (-65.7702, -48.5) ccw
  arc A14 (-65.7702, 28.5) -> (-51.624, 34.3619) centre (-65.7702, 48.5) ccw
  arc A15 (51.624, 34.3619) -> (65.7702, 28.5) centre (65.7702, 48.5) ccw
  arc A16 (65.7702, -28.5) -> (51.624, -34.3619) centre (65.7702, -48.5) ccw
  arc A17 (18.7124, -59) -> (32.8586, -53.1381) centre (18.7124, -39) ccw
  arc A18 (-32.8586, -53.1381) -> (-18.7124, -59) centre (-18.7124, -39) ccw
  arc A19 (-18.7124, 59) -> (-32.8586, 53.1381) centre (-18.7124, 39) ccw
  arc A20 (32.8586, 53.1381) -> (18.7124, 59) centre (18.7124, 39) ccw
  line L23 (42.1563, 22.5) -> (-42.6792, 22.5)
  arc A21 (-42.6792, 22.5) -> (-42.6792, 7.5) centre (-42.6792, 15) ccw
  line L24 (-42.6792, 7.5) -> (42.1563, 7.5)
  arc A22 (42.1563, 7.5) -> (42.1563, 22.5) centre (42.1563, 15) ccw
  line L25 (42.1563, 15) -> (-42.6792, 15) construction
  line L26 (-42.6792, -7.5) -> (42.1563, -7.5)
  arc A23 (42.1563, -22.5) -> (42.1563, -7.5) centre (42.1563, -15) ccw
  line L27 (42.1563, -22.5) -> (-42.6792, -22.5)
  arc A24 (-42.6792, -7.5) -> (-42.6792, -22.5) centre (-42.6792, -15) ccw
  line L28 (75, -15) -> (75, 15)
  arc A25 (75, 15) -> (65, 15) centre (70, 15) ccw
  line L29 (65, 15) -> (65, -15)
  arc A26 (65, -15) -> (75, -15) centre (70, -15) ccw
  line L30 (70, -15) -> (70, 15) construction
  line L31 (-75, -15) -> (-75, 15)
  line L32 (-65, 15) -> (-65, -15)
  arc A27 (-75, -15) -> (-65, -15) centre (-70, -15) ccw
  arc A28 (-65, 15) -> (-75, 15) centre (-70, 15) ccw
  point P0 (27, -59)
  dimension "d77" = 182
  dimension "d78" = 118
  dimension "d79" = 28.5
  dimension "d80" = 27
  dimension "d81" = 5
  dimension "d82" = 5
  dimension "d83" = 5
  dimension "d84" = 5
  dimension "d85" = 20
  dimension "d86" = 15
  dimension "d87" = 15
  dimension "d88" = 10
  constraint horizontal L5
  constraint perpendicular L5 L6
  constraint parallel L5 L7
  constraint parallel L6 L8
  constraint coincident L9 origin
  constraint coincident L10 origin
  constraint parallel L8 L11
  constraint perpendicular L11 L12
  constraint vertical L14
  constraint coincident L8 L11.start
  constraint horizontal L17
  constraint symmetric P0 L17 L20.end
  constraint coincident L11.end L12
  constraint tangent L12 A9
  constraint tangent L8 A9
  constraint tangent L8 A10
  constraint tangent L19 A10
  constraint tangent L16 A11
  constraint tangent L6 A11
  constraint tangent L6 A12
  constraint tangent L22 A12
  constraint tangent L16 A13
  constraint tangent L15 A13
  constraint tangent L21 A14
  constraint tangent L22 A14
  constraint equal A13 A14
  constraint tangent L18 A15
  constraint tangent L19 A15
  constraint equal A13 A15
  constraint tangent L12 A16
  constraint tangent L13 A16
  constraint equal A13 A16
  constraint coincident P0 L13
  constraint tangent L13 A17
  constraint tangent L7 A17
  constraint equal A13 A17
  constraint tangent L15 A18
  constraint tangent L7 A18
  constraint equal A13 A18
  constraint coincident L5.end L20
  constraint coincident L5.end L21
  constraint tangent L20 A19
  constraint tangent L21 A19
  constraint equal A13 A19
  constraint coincident L5 L20.end
  constraint coincident L20.end L18
  constraint tangent L5 A20
  constraint tangent L18 A20
  constraint equal A13 A20
  constraint tangent L23 A21
  constraint tangent A21 L24
  constraint parallel L23 L24
  constraint tangent L24 A22
  constraint tangent L23 A22
  constraint horizontal L25
  constraint symmetric L17 L23.start A23.start
  constraint symmetric L17 L23.end L27.end
  constraint symmetric L17 A21.end L26.start
  constraint symmetric L17 L24.end L26.end
  constraint symmetric L17 A21 A24
  constraint symmetric L17 A22 A23
  constraint tangent L28 A25
  constraint tangent A25 L29
  constraint parallel L28 L29
  constraint tangent L29 A26
  constraint tangent L28 A26
  constraint perpendicular L17 L30
  constraint symmetric L14 L28.start L31.start
  constraint symmetric L14 L28.end L31.end
  constraint symmetric L14 A25.end L32.start
  constraint symmetric L14 L29.end L32.end
  constraint symmetric L14 A25 A28
  constraint symmetric L14 A26 A27
  measures "d77" distance of L9.end L10.end
  measures "d78" distance of L10.start L9.end
  measures "d79" distance of L11.start L11.end
  measures "d80" horizontal distance of origin P0
  measures "d81" radius of A9
  measures "d82" radius of A10
  measures "d83" radius of A11
  measures "d84" radius of A12
  measures "d85" radius of A13
  measures "d86" diameter of A21
  measures "d87" distance of origin L25
  measures "d88" diameter of A25
extrude "Extrude8" add sketch "Sketch8" along normal blind 2 separate body contours L0 L1 L2 L3 L4 A0 L23 A21 | L5 L6 L7 L8 L11 L12 L13 L15 L16 L18 L19 L20 L21 L22 A9 A10 A11 A12 A13 A14 A15 A16 A17 A18 A19 A20 makes body 7
fillet "Fillet6" radius 10 4 edges at (-37.5858, 37.5858, 7) (-37.5858, -37.5858, 7) (37.5858, 37.5858, 7) (37.5858, -37.5858, 7) on bodies 3 4 5 6
equation "d4 = d3"
equation "d6 = d5"
equation "d8 = d7"
equation "d10 = d9"
equation "d79 = ( 57 / 2 ) * 1 mm"
named bodies: "top plate", "arm", "arm (1)", "arm (2)", "arm (1) (1)"
